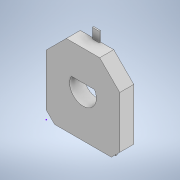
# Autodesk Inventor part: 3SR08_ポテンショメータ
Saved by Autodesk Inventor 2021 (Build 250183000, 183)
## iProperties
Created: 2021-04-20
Part Number: 3SR08_ポテンショメータ
Material: 一般
Document SubType Name: Modeling
Designer: ryusei
Density: 1 g/cm^3
Appearance: 既定
Author: ryusei
Autodesk Inventor part; units mm, degrees
ref_plane "YZ Plane" through (0, 0, 0) normal (1, 0, 0) x (0, 1, 0)
ref_plane "XZ Plane" through (0, 0, 0) normal (0, 1, 0) x (-1, 0, 0)
ref_plane "XY Plane" through (0, 0, 0) normal (0, 0, 1) x (1, 0, 0)
sketch "スケッチ1" plane through (0, 0, 0) normal (0, 0, 1) x (1, 0, 0)
  line L0 (0, 0) -> (11, 0)
  line L1 (11, 0) -> (11, 12)
  line L2 (11, 12) -> (0, 12)
  line L3 (0, 12) -> (0, 0)
  dimension "d0" = 11
  dimension "d1" = 12
  constraints: 8 end point, 2 parallel, 1 horizontal, 1 perpendicular
  measures "d0" distance between parallel lines of L1 L3
  measures "d1" distance between parallel lines of L0 L2
extrude "押し出し1" add sketch "スケッチ1" along normal blind 2.1
sketch "スケッチ2" plane through (0, 0, 2.1) normal (0, 0, 1) x (1, 0, 0)
  circle A0 centre (5.5, 6.5) radius 2
  line L0 (0, 12) -> (0, 0) projected
  line L1 (11, 12) -> (0, 12) projected
  line L2 (3.7679, 7.5) -> (7.2321, 7.5)
  dimension "d4" = 4
  dimension "d5" = 5.5
  dimension "d6" = 5.5
  dimension "d7" = 3
  constraints: 2 end point, 2 point on circle, 1 centre point, 1 horizontal
  measures "d4" diameter of A0
  measures "d5" distance from line of L0 A0.centre
  measures "d6" distance from line of L1 A0.centre
extrude "押し出し2" cut sketch "スケッチ2" against normal through all contours A0 L2 picked at (5.5553, 6.2487)
sketch "スケッチ3" plane through (0, 0, 2.1) normal (0, 0, 1) x (1, 0, 0)
  line L0 (0, 12) -> (0, 0) projected
  line L1 (0, 9) -> (3, 12)
  line L2 (11, 12) -> (0, 12) projected
  line L3 (0, 1) -> (1, 0)
  line L4 (0, 0) -> (11, 0) projected
  line L5 (5.5, 12) -> (5.5, 0)
  line L6 (11, 9) -> (8, 12)
  line L7 (11, 1) -> (10, 0)
  dimension "d10" = 45
  dimension "d12" = 1
  dimension "d13" = 3
  dimension "d14" = 1
  constraints: 10 end point, 4 point on line, 4 symmetric about line, 2 midpoint
  measures "d10" angle of L0 L1
  measures "d12" horizontal distance of L3.start L3.end
  measures "d13" horizontal distance of L1.start L1.end
  measures "d14" horizontal distance of L3.start L3.end
extrude "押し出し3" cut sketch "スケッチ3" against normal through all contours L2 L1 L0
sketch "スケッチ4" plane through (0, 0, 2.1) normal (0, 0, 1) x (1, 0, 0)
  line L0 (11, 12) -> (3, 12) projected
  line L1 (8, 12) -> (11, 9)
  line L2 (11, 0) -> (11, 12) projected
  point P0 (0, 0)
  dimension "d17" = 3
  dimension "d18" = 3
  constraints: 2 end point, 2 point on line
  measures "d17" horizontal distance of L1.start L1.end
  measures "d18" horizontal distance of L1.start L1.end
extrude "押し出し4" cut sketch "スケッチ4" against normal through all
sketch "スケッチ5" plane through (0, 0, 2.1) normal (0, 0, 1) x (1, 0, 0)
  line L0 (0, 9) -> (0, 0) projected
  line L1 (0, 1.25) -> (1.25, 0)
  line L2 (0, 0) -> (11, 0) projected
  dimension "d21" = 1.25
  dimension "d29" = 1.25
  constraints: 2 end point, 2 point on line
  measures "d21" horizontal distance of L1.start L1.end
  measures "d29" horizontal distance of L1.start L1.end
extrude "押し出し5" cut sketch "スケッチ5" against normal through all
sketch "スケッチ6" plane through (0, 0, 2.1) normal (0, 0, 1) x (1, 0, 0)
  line L0 (11, 0) -> (11, 9) projected
  line L1 (11, 1.25) -> (9.75, 0)
  line L2 (1.25, 0) -> (11, 0) projected
  point P0 (0, 0)
  dimension "d25" = 1.25
  dimension "d26" = 1.25
  constraints: 2 end point, 2 point on line
  measures "d25" horizontal distance of L1.start L1.end
  measures "d26" horizontal distance of L1.start L1.end
extrude "押し出し6" cut sketch "スケッチ6" against normal through all
sketch "スケッチ7" plane through (1.25, 0, 0) normal (0, -1, 0) x (1, 0, 0)
  point P0 (-1.25, 0)
sketch "スケッチ8" plane through (0, 0, 2.1) normal (0, 0, 1) x (1, 0, 0)
  point P0 (0, 0)
sketch "スケッチ9" plane through (0, 0, 2.1) normal (0, 0, 1) x (1, 0, 0)
  point P0 (0, 0)
sketch "スケッチ10" plane through (1.25, 0, 0) normal (0, -1, 0) x (1, 0, 0)
  line L0 (3.75, 0.2) -> (4.75, 0.2)
  line L1 (4.75, 0.2) -> (4.75, 0)
  line L2 (4.75, 0) -> (3.75, 0)
  line L3 (3.75, 0) -> (3.75, 0.2)
  line L4 (0, 0) -> (8.5, 0) projected
  line L5 (6.25, 0.2) -> (7.25, 0.2)
  line L6 (7.25, 0.2) -> (7.25, 0)
  line L7 (7.25, 0) -> (6.25, 0)
  line L8 (6.25, 0) -> (6.25, 0.2)
  line L9 (9.75, 2.1) -> (9.75, 0) projected
  point P0 (-1.25, 0)
  dimension "d31" = 1
  dimension "d36" = 0.2
  dimension "d37" = 1
  dimension "d38" = 2.5
  constraints: 16 end point, 4 parallel, 2 horizontal, 2 perpendicular, 1 point on line
  measures "d31" distance of L0.end L0.start
  measures "d36" distance between parallel lines of L4 L5
  measures "d37" distance of L5.end L5.start
  measures "d38" distance from line of L9 L6.end
sketch "スケッチ12" plane through (1.25, 0, 0) normal (0, -1, 0) x (1, 0, 0)
  line L0 (6.25, 2.1) -> (6.25, 0) projected
  line L1 (6.75, 0) -> (9.75, 0) projected
  line L2 (6.25, 0.2) -> (7.25, 0.2)
  line L3 (7.25, 0.2) -> (7.25, 0)
  line L4 (7.25, 0) -> (6.25, 0)
  line L5 (6.25, 0) -> (6.25, 0.2)
  point P0 (-1.25, 0)
  dimension "d34" = 1
  dimension "d35" = 0.2
  constraints: 8 end point, 2 parallel, 2 point on line, 1 horizontal, 1 perpendicular
  measures "d34" distance of L2.end L2.start
  measures "d35" distance from line of L1.start L2
extrude "押し出し7" add sketch "スケッチ10" along normal blind 1.4 contours L0 L1 L2 L3
extrude "押し出し8" add sketch "スケッチ12" along normal blind 1.4
sketch "スケッチ13" plane through (1.25, 0, 0) normal (0, -1, 0) x (1, 0, 0)
  line L0 (6.25, 0) -> (2.25, 0) projected
  line L1 (2.25, 0.2) -> (1.25, 0.2)
  line L2 (1.25, 0.2) -> (1.25, 0)
  line L3 (1.25, 0) -> (2.25, 0)
  line L4 (2.25, 0) -> (2.25, 0.2)
  line L5 (-1.25, 0) -> (-1.25, 2.1) projected
  point P0 (2.5179, 0)
  point P1 (5.9821, 0)
  dimension "d43" = 0.2
  dimension "d44" = 1
  dimension "d45" = 2.5
  constraints: 8 end point, 2 parallel, 1 horizontal, 1 perpendicular, 1 point on line
  measures "d43" distance between parallel lines of L0 L1
  measures "d44" distance between parallel lines of L4 L2
  measures "d45" distance between parallel lines of L5 L2
extrude "押し出し9" add sketch "スケッチ13" along normal blind 1.4
sketch "スケッチ14" plane through (3, 12, 2.1) normal (0, 1, 0) x (1, 0, 0)
  line L0 (2, 1.9) -> (3, 1.9) projected
  line L1 (0.5, 2.1) -> (4.5, 2.1) projected
  line L2 (2, 1.9) -> (3, 1.9)
  line L3 (3, 1.9) -> (3, 2.1)
  line L4 (3, 2.1) -> (2, 2.1)
  line L5 (2, 2.1) -> (2, 1.9)
  point P0 (-3, 2.1)
  point P1 (0.7679, 2.1)
  point P2 (4.2321, 2.1)
  dimension "d48" = 1
  constraints: 8 end point, 2 parallel, 1 horizontal, 1 perpendicular, 1 point on line
  measures "d48" distance from line of L3.end L5
extrude "押し出し10" add sketch "スケッチ14" along normal blind 1.5
